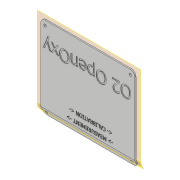
# Autodesk Inventor part: 03_Lid
Saved by Autodesk Inventor 2019.4 (Build 234330000, 330)
## iProperties
Created: 2021-06-05
Part Number: 03_Lid
Material: Generic
Document SubType Name: Modeling
Designer: diederichbenedict
Density: 1 g/cm^3
Appearance: Default
Author: diederichbenedict
Autodesk Inventor part; units mm, degrees
ref_plane "YZ Plane" through (0, 0, 0) normal (1, 0, 0) x (0, 1, 0)
ref_plane "XZ Plane" through (0, 0, 0) normal (0, 1, 0) x (-1, 0, 0)
ref_plane "XY Plane" through (0, 0, 0) normal (0, 0, 1) x (1, 0, 0)
ref_plane "Work Plane1" through (0, 0, 0) normal (0, 0, 1) x (1, 0, 0)
sketch "Sketch1" plane through (0, 0, 0) normal (0, 0, 1) x (1, 0, 0)
  ellipse E0 centre (-7.5, -84.2405) end of major axis (-7.5, -80.461) minor radius 1.5 projected
  ellipse E1 centre (-100.5, -84.2405) end of major axis (-100.5, -80.461) minor radius 1.5 projected
  ellipse E2 centre (-103, -7.7709) end of major axis (-103, -9.3506) minor radius 1.45 projected
  line L0 (-3, -61.2439) -> (-3, -12.7635) projected
  line L1 (-3, -61.2439) -> (-18, -61.2439) projected
  line L2 (-18, -90.5398) -> (-18, -61.2439) projected
  line L3 (0, -90.5398) -> (-18, -90.5398) projected
  line L4 (0, -7.7709) -> (0, -90.5398) projected
  ellipse E3 centre (-5, -7.7709) end of major axis (-5, -13.2183) minor radius 5 (0, -7.7709) -> (-5, -2.3235) ccw projected
  line L5 (-103, -2.3235) -> (-5, -2.3235) projected
  ellipse E4 centre (-103, -7.7709) end of major axis (-103, -13.2183) minor radius 5 (-103, -2.3235) -> (-108, -7.7709) ccw projected
  line L6 (-108, -90.5398) -> (-108, -7.7709) projected
  line L7 (-95, -90.5398) -> (-108, -90.5398) projected
  line L8 (-95, -61.2439) -> (-95, -90.5398) projected
  line L9 (-105, -61.2439) -> (-95, -61.2439) projected
  line L10 (-105, -12.7635) -> (-105, -61.2439) projected
  ellipse E5 centre (-103, -7.7709) end of major axis (-103, -13.2183) minor radius 5 (-105, -12.7635) -> (-98.4174, -5.5919) ccw projected
  line L11 (-9.5826, -5.5919) -> (-98.4174, -5.5919) projected
  ellipse E6 centre (-5, -7.7709) end of major axis (-5, -13.2183) minor radius 5 (-9.5826, -5.5919) -> (-3, -12.7635) ccw projected
  ellipse E7 centre (-5, -7.7709) end of major axis (-5, -9.3506) minor radius 1.45 projected
  line L12 (-18, -90.5398) -> (-95, -90.5398)
  point P0 (0, 0)
  constraints: 2 end point, 1 horizontal, 8 other
extrude "Extrusion1" add sketch "Sketch1" along normal blind 1.5 contours E0 | E1 | L1 L2 L12 L8 L9 L10 E5 L11 E6 L0 | L0 E6 L11 E5 L10 L9 L8 L7 L6 E4 L5 E3 L4 L3 L2 L1
ref_plane "Work Plane2" through (-54, -57.5226, 14.2761) normal (0, -0.3968725, 0.9178738) x (1, 0, 0)
sketch "Sketch2" plane through (-54, -57.5226, 14.2761) normal (0, -0.3968725, 0.9178738) x (1, 0, 0)
  circle A0 centre (49, -40) radius 1.45 projected
  circle A1 centre (-49, -40) radius 1.45 projected
  line L0 (-41, -35.9714) -> (-54, -35.9714) projected
  line L1 (-54, -40) -> (-54, -35.9714) projected
  arc A2 (-54, -40) -> (-49, -45) centre (-49, -40) ccw projected
  line L2 (49, -45) -> (-49, -45) projected
  arc A3 (49, -45) -> (54, -40) centre (49, -40) ccw projected
  line L3 (54, -35.9714) -> (54, -40) projected
  line L4 (54, -35.9714) -> (36, -35.9714) projected
  line L5 (36, -42) -> (36, -35.9714) projected
  line L6 (-41, -42) -> (36, -42) projected
  line L7 (-41, -35.9714) -> (-41, -42) projected
  line L8 (36, -35.9714) -> (-41, -35.9714)
  line L9 (-54, -35.9714) -> (54, -35.9714) projected
  line L10 (-54, 40) -> (-54, -35.9714) projected
  line L11 (54, -35.3761) -> (54, 40.5953) projected
  line L12 (-54, -35.9714) -> (54, -35.9714)
  line L13 (54, -35.9714) -> (54, -35.3761)
  line L14 (54, -35.3761) -> (-54, -35.3761)
  line L15 (-54, -35.3761) -> (-54, -35.9714)
  point P0 (54, 47.1327)
  constraints: 10 end point, 2 parallel, 1 collinear, 1 horizontal, 1 perpendicular
extrude "Extrusion2" add sketch "Sketch2" along normal up to surface (1.3768 mm away)
sketch "Sketch3" plane through (0, 0, 1.5) normal (0, 0, 1) x (1, 0, 0)
  ellipse E0 centre (-5, -7.7709) end of major axis (-5, -6.1911) minor radius 1.45 projected
  ellipse E1 centre (-103, -7.7709) end of major axis (-103, -6.1911) minor radius 1.45 projected
  line L0 (-108, -90.5398) -> (0, -90.5398) projected
  line L1 (0, -90.5398) -> (0, -7.7709) projected
  ellipse E2 centre (-5, -7.7709) end of major axis (-5, -13.2183) minor radius 5 (0, -7.7709) -> (-5, -2.3235) ccw projected
  line L2 (-5, -2.3235) -> (-103, -2.3235) projected
  ellipse E3 centre (-103, -7.7709) end of major axis (-103, -13.2183) minor radius 5 (-103, -2.3235) -> (-108, -7.7709) ccw projected
  line L3 (-108, -7.7709) -> (-108, -90.5398) projected
  line L4 (-3.7962, -33.7156) -> (-220.4518, -33.7156) construction
  line L5 (-220.4518, -33.7156) -> (-220.4518, 2.716) construction
  line L6 (-220.4518, 2.716) -> (-3.7962, 2.716) construction
  line L7 (-3.7962, 2.716) -> (-3.7962, -33.7156) construction
  line L8 (-24.8389, -87.8495) -> (-82.3672, -87.8495) construction
  line L9 (-82.3672, -87.8495) -> (-82.3672, -82.6215) construction
  line L10 (-82.3672, -82.6215) -> (-24.8389, -82.6215) construction
  line L11 (-24.8389, -82.6215) -> (-24.8389, -87.8495) construction
  line L12 (-25.7292, -78.9471) -> (-83.2575, -78.9471) construction
  line L13 (-83.2575, -78.9471) -> (-83.2575, -73.7191) construction
  line L14 (-83.2575, -73.7191) -> (-25.7292, -73.7191) construction
  line L15 (-25.7292, -73.7191) -> (-25.7292, -78.9471) construction
  spline S0 degree 2 poles (-14.4129, -31.9391) (-15.1575, -31.0668) (-15.9873, -28.5137) (-15.9873, -26.8754) knots 0 0 0 1 2 2 2
  spline S1 degree 2 poles (-15.9873, -26.8754) (-15.9873, -25.2798) (-15.1788, -22.6947) (-14.4129, -21.8224) knots 0 0 0 1 2 2 2
  spline S2 degree 2 poles (-14.4129, -21.8224) (-13.6044, -20.9076) (-11.4662, -20.0353) (-10.179, -20.0353) knots 0 0 0 1 2 2 2
  spline S3 degree 2 poles (-10.179, -20.0353) (-8.8492, -20.0353) (-6.7217, -20.9395) (-5.9451, -21.8224) knots 0 0 0 1 2 2 2
  spline S4 degree 2 poles (-5.9451, -21.8224) (-5.1898, -22.6947) (-4.3813, -25.2585) (-4.3813, -26.8754) knots 0 0 0 1 2 2 2
  spline S5 degree 2 poles (-4.3813, -26.8754) (-4.3813, -28.5243) (-5.2004, -31.0349) (-5.9557, -31.9391) knots 0 0 0 1 2 2 2
  spline S6 degree 2 poles (-5.9557, -31.9391) (-6.7217, -32.8114) (-8.8599, -33.7156) (-10.179, -33.7156) knots 0 0 0 1 2 2 2
  spline S7 degree 2 poles (-10.179, -33.7156) (-11.5194, -33.7156) (-13.6682, -32.7795) (-14.4129, -31.9391) knots 0 0 0 1 2 2 2
  spline S8 degree 2 poles (-14.1682, -26.8754) (-14.1682, -28.1733) (-13.6044, -30.1838) (-13.0938, -30.8434) knots 0 0 0 1 2 2 2
  spline S9 degree 2 poles (-13.0938, -30.8434) (-12.5725, -31.5242) (-11.1045, -32.205) (-10.1896, -32.205) knots 0 0 0 1 2 2 2
  spline S10 degree 2 poles (-10.1896, -32.205) (-9.2428, -32.205) (-7.8174, -31.5455) (-7.2748, -30.8434) knots 0 0 0 1 2 2 2
  spline S11 degree 2 poles (-7.2748, -30.8434) (-6.7536, -30.1732) (-6.2004, -28.152) (-6.2004, -26.8754) knots 0 0 0 1 2 2 2
  spline S12 degree 2 poles (-6.2004, -26.8754) (-6.2004, -24.2904) (-8.3705, -21.5458) (-10.1896, -21.5458) knots 0 0 0 1 2 2 2
  spline S13 degree 2 poles (-10.1896, -21.5458) (-12.0087, -21.5458) (-14.1682, -24.2904) (-14.1682, -26.8754) knots 0 0 0 1 2 2 2
  line L16 (-25.6252, -20.3118) -> (-17.5298, -20.3118)
  line L17 (-17.5298, -20.3118) -> (-17.5298, -22.1735)
  spline S14 degree 2 poles (-17.5298, -22.1735) (-18.4021, -22.9926) (-19.9552, -24.5138) (-20.6999, -25.3329) knots 0 0 0 1 2 2 2
  spline S15 degree 2 poles (-20.6999, -25.3329) (-22.1998, -26.9818) (-23.2955, -28.9605) (-23.2955, -30.0136) knots 0 0 0 1 2 2 2
  spline S16 degree 2 poles (-23.2955, -30.0136) (-23.2955, -30.5668) (-22.9551, -31.3966) (-22.6466, -31.6625) knots 0 0 0 1 2 2 2
  spline S17 degree 2 poles (-22.6466, -31.6625) (-22.3381, -31.9285) (-21.5296, -32.1944) (-21.0403, -32.1944) knots 0 0 0 1 2 2 2
  spline S18 degree 2 poles (-21.0403, -32.1944) (-20.5722, -32.1944) (-19.6148, -31.9604) (-19.1787, -31.7795) knots 0 0 0 1 2 2 2
  spline S19 degree 2 poles (-19.1787, -31.7795) (-18.8063, -31.6306) (-18.1149, -31.2051) (-17.9021, -31.0561) knots 0 0 0 1 2 2 2
  line L18 (-17.9021, -31.0561) -> (-17.8064, -31.0561)
  line L19 (-17.8064, -31.0561) -> (-17.8064, -32.9284)
  spline S20 degree 2 poles (-17.8064, -32.9284) (-18.3489, -33.1944) (-20.2956, -33.7156) (-21.168, -33.7156) knots 0 0 0 1 2 2 2
  spline S21 degree 2 poles (-21.168, -33.7156) (-23.0083, -33.7156) (-25.0827, -31.7689) (-25.0827, -30.1094) knots 0 0 0 1 2 2 2
  spline S22 degree 2 poles (-25.0827, -30.1094) (-25.0827, -29.3328) (-24.721, -28.035) (-24.4019, -27.4818) knots 0 0 0 1 2 2 2
  spline S23 degree 2 poles (-24.4019, -27.4818) (-24.0827, -26.9074) (-23.1572, -25.7797) (-22.6466, -25.2372) knots 0 0 0 1 2 2 2
  spline S24 degree 2 poles (-22.6466, -25.2372) (-21.8169, -24.333) (-19.785, -22.3969) (-19.1787, -21.8331) knots 0 0 0 1 2 2 2
  line L20 (-19.1787, -21.8331) -> (-25.6252, -21.8331)
  line L21 (-25.6252, -21.8331) -> (-25.6252, -20.3118)
  spline S25 degree 2 poles (-42.6778, -31.9391) (-43.4225, -31.0668) (-44.2523, -28.5137) (-44.2523, -26.8754) knots 0 0 0 1 2 2 2
  spline S26 degree 2 poles (-44.2523, -26.8754) (-44.2523, -25.2798) (-43.4438, -22.6947) (-42.6778, -21.8224) knots 0 0 0 1 2 2 2
  spline S27 degree 2 poles (-42.6778, -21.8224) (-41.8694, -20.9076) (-39.7311, -20.0353) (-38.4439, -20.0353) knots 0 0 0 1 2 2 2
  spline S28 degree 2 poles (-38.4439, -20.0353) (-37.1142, -20.0353) (-34.9866, -20.9395) (-34.2101, -21.8224) knots 0 0 0 1 2 2 2
  spline S29 degree 2 poles (-34.2101, -21.8224) (-33.4548, -22.6947) (-32.6463, -25.2585) (-32.6463, -26.8754) knots 0 0 0 1 2 2 2
  spline S30 degree 2 poles (-32.6463, -26.8754) (-32.6463, -28.5243) (-33.4654, -31.0349) (-34.2207, -31.9391) knots 0 0 0 1 2 2 2
  spline S31 degree 2 poles (-34.2207, -31.9391) (-34.9866, -32.8114) (-37.1248, -33.7156) (-38.4439, -33.7156) knots 0 0 0 1 2 2 2
  spline S32 degree 2 poles (-38.4439, -33.7156) (-39.7843, -33.7156) (-41.9332, -32.7795) (-42.6778, -31.9391) knots 0 0 0 1 2 2 2
  spline S33 degree 2 poles (-42.4332, -26.8754) (-42.4332, -28.1733) (-41.8694, -30.1838) (-41.3587, -30.8434) knots 0 0 0 1 2 2 2
  spline S34 degree 2 poles (-41.3587, -30.8434) (-40.8375, -31.5242) (-39.3694, -32.205) (-38.4546, -32.205) knots 0 0 0 1 2 2 2
  spline S35 degree 2 poles (-38.4546, -32.205) (-37.5078, -32.205) (-36.0823, -31.5455) (-35.5398, -30.8434) knots 0 0 0 1 2 2 2
  spline S36 degree 2 poles (-35.5398, -30.8434) (-35.0185, -30.1732) (-34.4654, -28.152) (-34.4654, -26.8754) knots 0 0 0 1 2 2 2
  spline S37 degree 2 poles (-34.4654, -26.8754) (-34.4654, -24.2904) (-36.6355, -21.5458) (-38.4546, -21.5458) knots 0 0 0 1 2 2 2
  spline S38 degree 2 poles (-38.4546, -21.5458) (-40.2737, -21.5458) (-42.4332, -24.2904) (-42.4332, -26.8754) knots 0 0 0 1 2 2 2
  spline S39 degree 2 poles (-54.2945, -25.5032) (-54.2945, -23.0352) (-51.9435, -20.1204) (-50.1457, -20.1204) knots 0 0 0 1 2 2 2
  spline S40 degree 2 poles (-50.1457, -20.1204) (-49.4116, -20.1204) (-48.284, -20.4608) (-47.6989, -20.8118) knots 0 0 0 1 2 2 2
  line L22 (-47.6989, -20.8118) -> (-47.6989, -16.6843)
  line L23 (-47.6989, -16.6843) -> (-46.0394, -16.6843)
  line L24 (-46.0394, -16.6843) -> (-46.0394, -30.1626)
  line L25 (-46.0394, -30.1626) -> (-47.6989, -30.1626)
  line L26 (-47.6989, -30.1626) -> (-47.6989, -29.1307)
  spline S41 degree 2 poles (-47.6989, -29.1307) (-48.3159, -29.6945) (-49.8265, -30.4391) (-50.7095, -30.4391) knots 0 0 0 1 2 2 2
  spline S42 degree 2 poles (-50.7095, -30.4391) (-52.4009, -30.4391) (-54.2945, -27.7584) (-54.2945, -25.5032) knots 0 0 0 1 2 2 2
  spline S43 degree 2 poles (-52.5817, -25.3117) (-52.5817, -27.0031) (-51.5073, -28.8647) (-50.3052, -28.8647) knots 0 0 0 1 2 2 2
  spline S44 degree 2 poles (-50.3052, -28.8647) (-49.6031, -28.8647) (-48.284, -28.2371) (-47.6989, -27.7478) knots 0 0 0 1 2 2 2
  line L27 (-47.6989, -27.7478) -> (-47.6989, -22.1522)
  spline S45 degree 2 poles (-47.6989, -22.1522) (-48.3479, -21.8437) (-49.2734, -21.6097) (-49.8691, -21.6097) knots 0 0 0 1 2 2 2
  spline S46 degree 2 poles (-49.8691, -21.6097) (-51.1563, -21.6097) (-52.5817, -23.5032) (-52.5817, -25.3117) knots 0 0 0 1 2 2 2
  spline S47 degree 2 poles (-60.2942, -20.0884) (-57.9326, -20.0884) (-55.337, -22.7373) (-55.337, -25.184) knots 0 0 0 1 2 2 2
  spline S48 degree 2 poles (-55.337, -25.184) (-55.337, -27.5882) (-57.8582, -30.4391) (-59.89, -30.4391) knots 0 0 0 1 2 2 2
  spline S49 degree 2 poles (-59.89, -30.4391) (-60.8049, -30.4391) (-62.2197, -29.9073) (-62.741, -29.3434) knots 0 0 0 1 2 2 2
  spline S50 degree 2 poles (-62.741, -29.3434) (-63.2729, -28.7796) (-63.8367, -27.152) (-63.8367, -25.9712) knots 0 0 0 1 2 2 2
  line L28 (-63.8367, -25.9712) -> (-63.8367, -25.067)
  line L29 (-63.8367, -25.067) -> (-57.0178, -25.067)
  spline S51 degree 2 poles (-57.0178, -25.067) (-57.0178, -23.3543) (-58.7411, -21.5352) (-60.273, -21.5352) knots 0 0 0 1 2 2 2
  spline S52 degree 2 poles (-60.273, -21.5352) (-60.8155, -21.5352) (-61.8687, -21.7799) (-62.2942, -21.9714) knots 0 0 0 1 2 2 2
  spline S53 degree 2 poles (-62.2942, -21.9714) (-62.741, -22.1841) (-63.358, -22.5564) (-63.5601, -22.7267) knots 0 0 0 1 2 2 2
  line L30 (-63.5601, -22.7267) -> (-63.6558, -22.7267)
  line L31 (-63.6558, -22.7267) -> (-63.6558, -20.9182)
  spline S54 degree 2 poles (-63.6558, -20.9182) (-63.3686, -20.8012) (-62.4963, -20.4608) (-62.1559, -20.365) knots 0 0 0 1 2 2 2
  spline S55 degree 2 poles (-62.1559, -20.365) (-61.6772, -20.2267) (-60.89, -20.0884) (-60.2942, -20.0884) knots 0 0 0 1 2 2 2
  spline S56 degree 2 poles (-62.2197, -26.3329) (-62.1984, -27.0031) (-61.9218, -27.9818) (-61.6559, -28.3116) knots 0 0 0 1 2 2 2
  spline S57 degree 2 poles (-61.6559, -28.3116) (-61.3687, -28.6839) (-60.4645, -29.0775) (-59.7943, -29.0775) knots 0 0 0 1 2 2 2
  spline S58 degree 2 poles (-59.7943, -29.0775) (-59.1347, -29.0775) (-58.2092, -28.6839) (-57.8262, -28.3009) knots 0 0 0 1 2 2 2
  spline S59 degree 2 poles (-57.8262, -28.3009) (-57.4539, -27.9073) (-57.071, -26.9605) (-57.0178, -26.3329) knots 0 0 0 1 2 2 2
  line L32 (-57.0178, -26.3329) -> (-62.2197, -26.3329)
  line L33 (-73.2512, -20.3118) -> (-71.5917, -20.3118)
  line L34 (-71.5917, -20.3118) -> (-71.5917, -25.9287)
  spline S60 degree 2 poles (-71.5917, -25.9287) (-71.5917, -26.6095) (-71.4641, -27.7797) (-71.2726, -28.1307) knots 0 0 0 1 2 2 2
  spline S61 degree 2 poles (-71.2726, -28.1307) (-71.0705, -28.503) (-70.3471, -28.8647) (-69.7301, -28.8647) knots 0 0 0 1 2 2 2
  spline S62 degree 2 poles (-69.7301, -28.8647) (-69.1131, -28.8647) (-67.8046, -28.2052) (-67.177, -27.6733) knots 0 0 0 1 2 2 2
  line L35 (-67.177, -27.6733) -> (-67.177, -20.3118)
  line L36 (-67.177, -20.3118) -> (-65.5175, -20.3118)
  line L37 (-65.5175, -20.3118) -> (-65.5175, -30.1626)
  line L38 (-65.5175, -30.1626) -> (-67.177, -30.1626)
  line L39 (-67.177, -30.1626) -> (-67.177, -29.0669)
  spline S63 degree 2 poles (-67.177, -29.0669) (-67.9216, -29.737) (-69.3578, -30.4391) (-70.1662, -30.4391) knots 0 0 0 1 2 2 2
  spline S64 degree 2 poles (-70.1662, -30.4391) (-71.613, -30.4391) (-73.2512, -28.5243) (-73.2512, -26.7052) knots 0 0 0 1 2 2 2
  line L40 (-73.2512, -26.7052) -> (-73.2512, -20.3118)
  spline S65 degree 2 poles (-84.9955, -31.9391) (-85.7402, -31.0668) (-86.5699, -28.5137) (-86.5699, -26.8754) knots 0 0 0 1 2 2 2
  spline S66 degree 2 poles (-86.5699, -26.8754) (-86.5699, -25.2798) (-85.7614, -22.6947) (-84.9955, -21.8224) knots 0 0 0 1 2 2 2
  spline S67 degree 2 poles (-84.9955, -21.8224) (-84.187, -20.9076) (-82.0488, -20.0353) (-80.7616, -20.0353) knots 0 0 0 1 2 2 2
  spline S68 degree 2 poles (-80.7616, -20.0353) (-79.4319, -20.0353) (-77.3043, -20.9395) (-76.5277, -21.8224) knots 0 0 0 1 2 2 2
  spline S69 degree 2 poles (-76.5277, -21.8224) (-75.7724, -22.6947) (-74.9639, -25.2585) (-74.9639, -26.8754) knots 0 0 0 1 2 2 2
  spline S70 degree 2 poles (-74.9639, -26.8754) (-74.9639, -28.5243) (-75.7831, -31.0349) (-76.5384, -31.9391) knots 0 0 0 1 2 2 2
  spline S71 degree 2 poles (-76.5384, -31.9391) (-77.3043, -32.8114) (-79.4425, -33.7156) (-80.7616, -33.7156) knots 0 0 0 1 2 2 2
  spline S72 degree 2 poles (-80.7616, -33.7156) (-82.102, -33.7156) (-84.2509, -32.7795) (-84.9955, -31.9391) knots 0 0 0 1 2 2 2
  spline S73 degree 2 poles (-84.7508, -26.8754) (-84.7508, -28.1733) (-84.187, -30.1838) (-83.6764, -30.8434) knots 0 0 0 1 2 2 2
  spline S74 degree 2 poles (-83.6764, -30.8434) (-83.1551, -31.5242) (-81.6871, -32.205) (-80.7723, -32.205) knots 0 0 0 1 2 2 2
  spline S75 degree 2 poles (-80.7723, -32.205) (-79.8255, -32.205) (-78.4, -31.5455) (-77.8575, -30.8434) knots 0 0 0 1 2 2 2
  spline S76 degree 2 poles (-77.8575, -30.8434) (-77.3362, -30.1732) (-76.783, -28.152) (-76.783, -26.8754) knots 0 0 0 1 2 2 2
  spline S77 degree 2 poles (-76.783, -26.8754) (-76.783, -24.2904) (-78.9532, -21.5458) (-80.7723, -21.5458) knots 0 0 0 1 2 2 2
  spline S78 degree 2 poles (-80.7723, -21.5458) (-82.5913, -21.5458) (-84.7508, -24.2904) (-84.7508, -26.8754) knots 0 0 0 1 2 2 2
  line L41 (-96.0058, -20.3118) -> (-93.9739, -20.3118)
  line L42 (-93.9739, -20.3118) -> (-91.5804, -24.0138)
  line L43 (-91.5804, -24.0138) -> (-89.123, -20.3118)
  line L44 (-89.123, -20.3118) -> (-87.2401, -20.3118)
  line L45 (-87.2401, -20.3118) -> (-90.6549, -25.1947)
  line L46 (-90.6549, -25.1947) -> (-87.272, -30.1626)
  line L47 (-87.272, -30.1626) -> (-89.3039, -30.1626)
  line L48 (-89.3039, -30.1626) -> (-91.6868, -26.4925)
  line L49 (-91.6868, -26.4925) -> (-94.1228, -30.1626)
  line L50 (-94.1228, -30.1626) -> (-96.0058, -30.1626)
  line L51 (-96.0058, -30.1626) -> (-92.6123, -25.301)
  line L52 (-92.6123, -25.301) -> (-96.0058, -20.3118)
  line L53 (-105.0267, -30.1626) -> (-99.729, -16.6843)
  line L54 (-99.729, -16.6843) -> (-97.9525, -16.6843)
  line L55 (-97.9525, -16.6843) -> (-99.7184, -20.7906)
  line L56 (-99.7184, -20.7906) -> (-96.1441, -30.1626)
  line L57 (-96.1441, -30.1626) -> (-97.9312, -30.1626)
  line L58 (-97.9312, -30.1626) -> (-100.6226, -22.8649)
  line L59 (-100.6226, -22.8649) -> (-103.3034, -30.1626)
  line L60 (-103.3034, -30.1626) -> (-105.0267, -30.1626)
  line L61 (-29.1554, -75.0735) -> (-26.2705, -76.4512)
  line L62 (-26.2705, -76.4512) -> (-26.2705, -76.7721)
  line L63 (-26.2705, -76.7721) -> (-29.1554, -78.1497)
  line L64 (-29.1554, -78.1497) -> (-29.1554, -77.6732)
  line L65 (-29.1554, -77.6732) -> (-26.9188, -76.6132)
  line L66 (-26.9188, -76.6132) -> (-29.1554, -75.55)
  line L67 (-29.1554, -75.55) -> (-29.1554, -75.0735)
  line L68 (-31.4893, -76.3701) -> (-29.9755, -76.3701)
  line L69 (-29.9755, -76.3701) -> (-29.9755, -76.8564)
  line L70 (-29.9755, -76.8564) -> (-31.4893, -76.8564)
  line L71 (-31.4893, -76.8564) -> (-31.4893, -76.3701)
  spline S79 degree 2 poles (-35.4147, -74.7915) (-35.0257, -74.7915) (-34.3677, -75.0541) (-34.1279, -75.3167) knots 0 0 0 1 2 2 2
  spline S80 degree 2 poles (-34.1279, -75.3167) (-33.888, -75.576) (-33.6254, -76.3539) (-33.6254, -76.8596) knots 0 0 0 1 2 2 2
  spline S81 degree 2 poles (-33.6254, -76.8596) (-33.6254, -77.362) (-33.8815, -78.1076) (-34.1246, -78.3831) knots 0 0 0 1 2 2 2
  spline S82 degree 2 poles (-34.1246, -78.3831) (-34.3645, -78.6521) (-35.0193, -78.9342) (-35.4245, -78.9342) knots 0 0 0 1 2 2 2
  spline S83 degree 2 poles (-35.4245, -78.9342) (-35.6254, -78.9342) (-35.9787, -78.8758) (-36.1279, -78.8304) knots 0 0 0 1 2 2 2
  spline S84 degree 2 poles (-36.1279, -78.8304) (-36.2575, -78.7883) (-36.5266, -78.6684) (-36.6595, -78.597) knots 0 0 0 1 2 2 2
  line L72 (-36.6595, -78.597) -> (-36.6595, -77.9552)
  line L73 (-36.6595, -77.9552) -> (-36.6173, -77.9552)
  spline S85 degree 2 poles (-36.6173, -77.9552) (-36.546, -78.0201) (-36.3256, -78.2016) (-36.1668, -78.2891) knots 0 0 0 1 2 2 2
  spline S86 degree 2 poles (-36.1668, -78.2891) (-36.0144, -78.3734) (-35.6546, -78.4803) (-35.4212, -78.4803) knots 0 0 0 1 2 2 2
  spline S87 degree 2 poles (-35.4212, -78.4803) (-35.1651, -78.4803) (-34.7081, -78.2697) (-34.5363, -78.0687) knots 0 0 0 1 2 2 2
  spline S88 degree 2 poles (-34.5363, -78.0687) (-34.3677, -77.8645) (-34.1797, -77.2453) (-34.1797, -76.8596) knots 0 0 0 1 2 2 2
  spline S89 degree 2 poles (-34.1797, -76.8596) (-34.1797, -76.4479) (-34.3774, -75.8547) (-34.5492, -75.6505) knots 0 0 0 1 2 2 2
  spline S90 degree 2 poles (-34.5492, -75.6505) (-34.7178, -75.4528) (-35.1684, -75.2518) (-35.4212, -75.2518) knots 0 0 0 1 2 2 2
  spline S91 degree 2 poles (-35.4212, -75.2518) (-35.6514, -75.2518) (-36.0436, -75.3653) (-36.1959, -75.4496) knots 0 0 0 1 2 2 2
  spline S92 degree 2 poles (-36.1959, -75.4496) (-36.3418, -75.5338) (-36.559, -75.7089) (-36.6206, -75.7705) knots 0 0 0 1 2 2 2
  line L74 (-36.6206, -75.7705) -> (-36.6595, -75.7705)
  line L75 (-36.6595, -75.7705) -> (-36.6595, -75.1351)
  spline S93 degree 2 poles (-36.6595, -75.1351) (-36.5266, -75.0735) (-36.2932, -74.9601) (-36.1279, -74.9082) knots 0 0 0 1 2 2 2
  spline S94 degree 2 poles (-36.1279, -74.9082) (-35.9528, -74.8499) (-35.6546, -74.7915) (-35.4147, -74.7915) knots 0 0 0 1 2 2 2
  line L76 (-36.7243, -74.8628) -> (-38.0727, -78.8628)
  line L77 (-38.0727, -78.8628) -> (-38.7275, -78.8628)
  line L78 (-38.7275, -78.8628) -> (-40.076, -74.8628)
  line L79 (-40.076, -74.8628) -> (-39.5152, -74.8628)
  line L80 (-39.5152, -74.8628) -> (-39.1522, -75.9812)
  line L81 (-39.1522, -75.9812) -> (-37.6254, -75.9812)
  line L82 (-37.6254, -75.9812) -> (-37.2624, -74.8628)
  line L83 (-37.2624, -74.8628) -> (-36.7243, -74.8628)
  line L84 (-39.0063, -76.435) -> (-38.3872, -78.3183)
  line L85 (-38.3872, -78.3183) -> (-37.7713, -76.435)
  line L86 (-37.7713, -76.435) -> (-39.0063, -76.435)
  line L87 (-42.7729, -74.8628) -> (-40.4552, -74.8628)
  line L88 (-40.4552, -74.8628) -> (-40.4552, -78.8628)
  line L89 (-40.4552, -78.8628) -> (-40.9869, -78.8628)
  line L90 (-40.9869, -78.8628) -> (-40.9869, -75.3361)
  line L91 (-40.9869, -75.3361) -> (-42.7729, -75.3361)
  line L92 (-42.7729, -75.3361) -> (-42.7729, -74.8628)
  line L93 (-44.5849, -74.8628) -> (-43.0355, -74.8628)
  line L94 (-43.0355, -74.8628) -> (-43.0355, -75.2713)
  line L95 (-43.0355, -75.2713) -> (-43.5444, -75.2713)
  line L96 (-43.5444, -75.2713) -> (-43.5444, -78.4544)
  line L97 (-43.5444, -78.4544) -> (-43.0355, -78.4544)
  line L98 (-43.0355, -78.4544) -> (-43.0355, -78.8628)
  line L99 (-43.0355, -78.8628) -> (-44.5849, -78.8628)
  line L100 (-44.5849, -78.8628) -> (-44.5849, -78.4544)
  line L101 (-44.5849, -78.4544) -> (-44.076, -78.4544)
  line L102 (-44.076, -78.4544) -> (-44.076, -75.2713)
  line L103 (-44.076, -75.2713) -> (-44.5849, -75.2713)
  line L104 (-44.5849, -75.2713) -> (-44.5849, -74.8628)
  spline S95 degree 2 poles (-47.9561, -76.0914) (-47.9561, -75.7932) (-47.7292, -75.3361) (-47.5411, -75.187) knots 0 0 0 1 2 2 2
  spline S96 degree 2 poles (-47.5411, -75.187) (-47.3142, -75.012) (-46.7988, -74.8628) (-46.3904, -74.8628) knots 0 0 0 1 2 2 2
  line L105 (-46.3904, -74.8628) -> (-45.2429, -74.8628)
  line L106 (-45.2429, -74.8628) -> (-45.2429, -78.8628)
  line L107 (-45.2429, -78.8628) -> (-46.3029, -78.8628)
  spline S97 degree 2 poles (-46.3029, -78.8628) (-46.7308, -78.8628) (-47.1586, -78.8077) (-47.3531, -78.7008) knots 0 0 0 1 2 2 2
  spline S98 degree 2 poles (-47.3531, -78.7008) (-47.5703, -78.5873) (-47.768, -78.2145) (-47.768, -77.9617) knots 0 0 0 1 2 2 2
  spline S99 degree 2 poles (-47.768, -77.9617) (-47.768, -77.6797) (-47.4698, -77.2324) (-47.2073, -77.106) knots 0 0 0 1 2 2 2
  line L108 (-47.2073, -77.106) -> (-47.2073, -77.0865)
  spline S100 degree 2 poles (-47.2073, -77.0865) (-47.5638, -76.9893) (-47.9561, -76.4739) (-47.9561, -76.0914) knots 0 0 0 1 2 2 2
  spline S101 degree 2 poles (-47.4018, -76.0687) (-47.4018, -76.2956) (-47.2721, -76.5873) (-47.0776, -76.691) knots 0 0 0 1 2 2 2
  spline S102 degree 2 poles (-47.0776, -76.691) (-46.9512, -76.7559) (-46.653, -76.7948) (-46.3774, -76.7948) knots 0 0 0 1 2 2 2
  line L109 (-46.3774, -76.7948) -> (-45.7745, -76.7948)
  line L110 (-45.7745, -76.7948) -> (-45.7745, -75.3167)
  line L111 (-45.7745, -75.3167) -> (-46.2057, -75.3167)
  spline S103 degree 2 poles (-46.2057, -75.3167) (-46.5557, -75.3167) (-46.9577, -75.3815) (-47.1133, -75.4852) knots 0 0 0 1 2 2 2
  spline S104 degree 2 poles (-47.1133, -75.4852) (-47.2624, -75.5922) (-47.4018, -75.858) (-47.4018, -76.0687) knots 0 0 0 1 2 2 2
  spline S105 degree 2 poles (-47.2138, -77.8872) (-47.2138, -78.0298) (-47.1165, -78.2437) (-47.0095, -78.3053) knots 0 0 0 1 2 2 2
  spline S106 degree 2 poles (-47.0095, -78.3053) (-46.8799, -78.3766) (-46.5655, -78.409) (-46.2834, -78.409) knots 0 0 0 1 2 2 2
  line L112 (-46.2834, -78.409) -> (-45.7745, -78.409)
  line L113 (-45.7745, -78.409) -> (-45.7745, -77.2389)
  line L114 (-45.7745, -77.2389) -> (-46.3774, -77.2389)
  spline S107 degree 2 poles (-46.3774, -77.2389) (-46.627, -77.2389) (-46.8637, -77.2907) (-46.9901, -77.3718) knots 0 0 0 1 2 2 2
  spline S108 degree 2 poles (-46.9901, -77.3718) (-47.1133, -77.4496) (-47.2138, -77.6991) (-47.2138, -77.8872) knots 0 0 0 1 2 2 2
  line L115 (-51.58, -74.8628) -> (-50.8896, -74.8628)
  line L116 (-50.8896, -74.8628) -> (-49.6254, -76.4544)
  line L117 (-49.6254, -76.4544) -> (-49.016, -76.4544)
  line L118 (-49.016, -76.4544) -> (-49.016, -74.8628)
  line L119 (-49.016, -74.8628) -> (-48.4844, -74.8628)
  line L120 (-48.4844, -74.8628) -> (-48.4844, -78.8628)
  line L121 (-48.4844, -78.8628) -> (-49.5152, -78.8628)
  spline S109 degree 2 poles (-49.5152, -78.8628) (-49.8588, -78.8628) (-50.3223, -78.7883) (-50.533, -78.6521) knots 0 0 0 1 2 2 2
  spline S110 degree 2 poles (-50.533, -78.6521) (-50.7437, -78.516) (-50.9869, -78.0914) (-50.9869, -77.7769) knots 0 0 0 1 2 2 2
  spline S111 degree 2 poles (-50.9869, -77.7769) (-50.9869, -77.3393) (-50.5395, -76.7461) (-50.157, -76.6035) knots 0 0 0 1 2 2 2
  line L122 (-50.157, -76.6035) -> (-51.58, -74.8628)
  spline S112 degree 2 poles (-50.4326, -77.7348) (-50.4326, -77.9098) (-50.3094, -78.1789) (-50.1797, -78.2664) knots 0 0 0 1 2 2 2
  spline S113 degree 2 poles (-50.1797, -78.2664) (-50.0663, -78.341) (-49.7648, -78.4026) (-49.5444, -78.4026) knots 0 0 0 1 2 2 2
  line L123 (-49.5444, -78.4026) -> (-49.016, -78.4026)
  line L124 (-49.016, -78.4026) -> (-49.016, -76.8985)
  line L125 (-49.016, -76.8985) -> (-49.4828, -76.8985)
  spline S114 degree 2 poles (-49.4828, -76.8985) (-49.7129, -76.8985) (-50.0792, -76.9795) (-50.2057, -77.106) knots 0 0 0 1 2 2 2
  spline S115 degree 2 poles (-50.2057, -77.106) (-50.3223, -77.2162) (-50.4326, -77.5273) (-50.4326, -77.7348) knots 0 0 0 1 2 2 2
  line L126 (-51.4666, -74.8628) -> (-52.8151, -78.8628)
  line L127 (-52.8151, -78.8628) -> (-53.4698, -78.8628)
  line L128 (-53.4698, -78.8628) -> (-54.8183, -74.8628)
  line L129 (-54.8183, -74.8628) -> (-54.2575, -74.8628)
  line L130 (-54.2575, -74.8628) -> (-53.8945, -75.9812)
  line L131 (-53.8945, -75.9812) -> (-52.3677, -75.9812)
  line L132 (-52.3677, -75.9812) -> (-52.0047, -74.8628)
  line L133 (-52.0047, -74.8628) -> (-51.4666, -74.8628)
  line L134 (-53.7486, -76.435) -> (-53.1295, -78.3183)
  line L135 (-53.1295, -78.3183) -> (-52.5136, -76.435)
  line L136 (-52.5136, -76.435) -> (-53.7486, -76.435)
  line L137 (-56.1311, -74.8628) -> (-56.1311, -78.3896)
  line L138 (-56.1311, -78.3896) -> (-54.7891, -78.3896)
  line L139 (-54.7891, -78.3896) -> (-54.7891, -78.8628)
  line L140 (-54.7891, -78.8628) -> (-58.0047, -78.8628)
  line L141 (-58.0047, -78.8628) -> (-58.0047, -78.3896)
  line L142 (-58.0047, -78.3896) -> (-56.6627, -78.3896)
  line L143 (-56.6627, -78.3896) -> (-56.6627, -74.8628)
  line L144 (-56.6627, -74.8628) -> (-56.1311, -74.8628)
  line L145 (-59.8037, -74.8628) -> (-58.2543, -74.8628)
  line L146 (-58.2543, -74.8628) -> (-58.2543, -75.2713)
  line L147 (-58.2543, -75.2713) -> (-58.7632, -75.2713)
  line L148 (-58.7632, -75.2713) -> (-58.7632, -78.4544)
  line L149 (-58.7632, -78.4544) -> (-58.2543, -78.4544)
  line L150 (-58.2543, -78.4544) -> (-58.2543, -78.8628)
  line L151 (-58.2543, -78.8628) -> (-59.8037, -78.8628)
  line L152 (-59.8037, -78.8628) -> (-59.8037, -78.4544)
  line L153 (-59.8037, -78.4544) -> (-59.2948, -78.4544)
  line L154 (-59.2948, -78.4544) -> (-59.2948, -75.2713)
  line L155 (-59.2948, -75.2713) -> (-59.8037, -75.2713)
  line L156 (-59.8037, -75.2713) -> (-59.8037, -74.8628)
  spline S116 degree 2 poles (-63.2916, -78.4058) (-63.5185, -78.14) (-63.7713, -77.362) (-63.7713, -76.8628) knots 0 0 0 1 2 2 2
  spline S117 degree 2 poles (-63.7713, -76.8628) (-63.7713, -76.3766) (-63.5249, -75.5889) (-63.2916, -75.3231) knots 0 0 0 1 2 2 2
  spline S118 degree 2 poles (-63.2916, -75.3231) (-63.0452, -75.0444) (-62.3937, -74.7786) (-62.0014, -74.7786) knots 0 0 0 1 2 2 2
  spline S119 degree 2 poles (-62.0014, -74.7786) (-61.5963, -74.7786) (-60.948, -75.0541) (-60.7113, -75.3231) knots 0 0 0 1 2 2 2
  spline S120 degree 2 poles (-60.7113, -75.3231) (-60.4812, -75.5889) (-60.2348, -76.3701) (-60.2348, -76.8628) knots 0 0 0 1 2 2 2
  spline S121 degree 2 poles (-60.2348, -76.8628) (-60.2348, -77.3653) (-60.4844, -78.1303) (-60.7146, -78.4058) knots 0 0 0 1 2 2 2
  spline S122 degree 2 poles (-60.7146, -78.4058) (-60.948, -78.6716) (-61.5995, -78.9471) (-62.0014, -78.9471) knots 0 0 0 1 2 2 2
  spline S123 degree 2 poles (-62.0014, -78.9471) (-62.4099, -78.9471) (-63.0646, -78.6619) (-63.2916, -78.4058) knots 0 0 0 1 2 2 2
  spline S124 degree 2 poles (-63.217, -76.8628) (-63.217, -77.2583) (-63.0452, -77.8709) (-62.8896, -78.0719) knots 0 0 0 1 2 2 2
  spline S125 degree 2 poles (-62.8896, -78.0719) (-62.7308, -78.2794) (-62.2834, -78.4868) (-62.0047, -78.4868) knots 0 0 0 1 2 2 2
  spline S126 degree 2 poles (-62.0047, -78.4868) (-61.7162, -78.4868) (-61.2818, -78.2859) (-61.1165, -78.0719) knots 0 0 0 1 2 2 2
  spline S127 degree 2 poles (-61.1165, -78.0719) (-60.9577, -77.8677) (-60.7891, -77.2518) (-60.7891, -76.8628) knots 0 0 0 1 2 2 2
  spline S128 degree 2 poles (-60.7891, -76.8628) (-60.7891, -76.0752) (-61.4504, -75.2389) (-62.0047, -75.2389) knots 0 0 0 1 2 2 2
  spline S129 degree 2 poles (-62.0047, -75.2389) (-62.559, -75.2389) (-63.217, -76.0752) (-63.217, -76.8628) knots 0 0 0 1 2 2 2
  line L157 (-67.217, -74.8628) -> (-66.6206, -74.8628)
  line L158 (-66.6206, -74.8628) -> (-64.8507, -78.3118)
  line L159 (-64.8507, -78.3118) -> (-64.8507, -74.8628)
  line L160 (-64.8507, -74.8628) -> (-64.3548, -74.8628)
  line L161 (-64.3548, -74.8628) -> (-64.3548, -78.8628)
  line L162 (-64.3548, -78.8628) -> (-65.11, -78.8628)
  line L163 (-65.11, -78.8628) -> (-66.721, -75.6959)
  line L164 (-66.721, -75.6959) -> (-66.721, -78.8628)
  line L165 (-66.721, -78.8628) -> (-67.217, -78.8628)
  line L166 (-67.217, -78.8628) -> (-67.217, -74.8628)
  line L167 (-72.7664, -75.0735) -> (-69.8815, -76.4512)
  line L168 (-69.8815, -76.4512) -> (-69.8815, -76.7721)
  line L169 (-69.8815, -76.7721) -> (-72.7664, -78.1497)
  line L170 (-72.7664, -78.1497) -> (-72.7664, -77.6732)
  line L171 (-72.7664, -77.6732) -> (-70.5298, -76.6132)
  line L172 (-70.5298, -76.6132) -> (-72.7664, -75.55)
  line L173 (-72.7664, -75.55) -> (-72.7664, -75.0735)
  line L174 (-75.1003, -76.3701) -> (-73.5865, -76.3701)
  line L175 (-73.5865, -76.3701) -> (-73.5865, -76.8564)
  line L176 (-73.5865, -76.8564) -> (-75.1003, -76.8564)
  line L177 (-75.1003, -76.8564) -> (-75.1003, -76.3701)
  line L178 (-26.5958, -85.2855) -> (-25.082, -85.2855)
  line L179 (-25.082, -85.2855) -> (-25.082, -85.7717)
  line L180 (-25.082, -85.7717) -> (-26.5958, -85.7717)
  line L181 (-26.5958, -85.7717) -> (-26.5958, -85.2855)
  line L182 (-30.2976, -85.3665) -> (-27.4127, -83.9889)
  line L183 (-27.4127, -83.9889) -> (-27.4127, -84.4654)
  line L184 (-27.4127, -84.4654) -> (-29.6493, -85.5286)
  line L185 (-29.6493, -85.5286) -> (-27.4127, -86.5886)
  line L186 (-27.4127, -86.5886) -> (-27.4127, -87.0651)
  line L187 (-27.4127, -87.0651) -> (-30.2976, -85.6874)
  line L188 (-30.2976, -85.6874) -> (-30.2976, -85.3665)
  line L189 (-36.3916, -83.7782) -> (-35.86, -83.7782)
  line L190 (-35.86, -83.7782) -> (-35.86, -87.2239)
  line L191 (-35.86, -87.2239) -> (-34.8162, -84.8803)
  line L192 (-34.8162, -84.8803) -> (-34.4921, -84.8803)
  line L193 (-34.4921, -84.8803) -> (-33.458, -87.2239)
  line L194 (-33.458, -87.2239) -> (-33.458, -83.7782)
  line L195 (-33.458, -83.7782) -> (-32.9621, -83.7782)
  line L196 (-32.9621, -83.7782) -> (-32.9621, -87.7782)
  line L197 (-32.9621, -87.7782) -> (-33.6882, -87.7782)
  line L198 (-33.6882, -87.7782) -> (-34.6866, -85.5513)
  line L199 (-34.6866, -85.5513) -> (-35.6525, -87.7782)
  line L200 (-35.6525, -87.7782) -> (-36.3916, -87.7782)
  line L201 (-36.3916, -87.7782) -> (-36.3916, -83.7782)
  line L202 (-37.202, -83.7782) -> (-37.202, -87.7782)
  line L203 (-37.202, -87.7782) -> (-39.7044, -87.7782)
  line L204 (-39.7044, -87.7782) -> (-39.7044, -87.305)
  line L205 (-39.7044, -87.305) -> (-37.7336, -87.305)
  line L206 (-37.7336, -87.305) -> (-37.7336, -86.2093)
  line L207 (-37.7336, -86.2093) -> (-39.5715, -86.2093)
  line L208 (-39.5715, -86.2093) -> (-39.5715, -85.7361)
  line L209 (-39.5715, -85.7361) -> (-37.7336, -85.7361)
  line L210 (-37.7336, -85.7361) -> (-37.7336, -84.2515)
  line L211 (-37.7336, -84.2515) -> (-39.7044, -84.2515)
  line L212 (-39.7044, -84.2515) -> (-39.7044, -83.7782)
  line L213 (-39.7044, -83.7782) -> (-37.202, -83.7782)
  line L214 (-39.8567, -83.7782) -> (-41.2052, -87.7782)
  line L215 (-41.2052, -87.7782) -> (-41.86, -87.7782)
  line L216 (-41.86, -87.7782) -> (-43.2084, -83.7782)
  line L217 (-43.2084, -83.7782) -> (-42.6477, -83.7782)
  line L218 (-42.6477, -83.7782) -> (-42.2846, -84.8965)
  line L219 (-42.2846, -84.8965) -> (-40.7579, -84.8965)
  line L220 (-40.7579, -84.8965) -> (-40.3948, -83.7782)
  line L221 (-40.3948, -83.7782) -> (-39.8567, -83.7782)
  line L222 (-42.1387, -85.3503) -> (-41.5196, -87.2336)
  line L223 (-41.5196, -87.2336) -> (-40.9037, -85.3503)
  line L224 (-40.9037, -85.3503) -> (-42.1387, -85.3503)
  spline S130 degree 2 poles (-44.7028, -83.7069) (-44.2684, -83.7069) (-43.659, -83.8884) (-43.39, -84.0181) knots 0 0 0 1 2 2 2
  line L225 (-43.39, -84.0181) -> (-43.39, -84.6858)
  line L226 (-43.39, -84.6858) -> (-43.4289, -84.6858)
  spline S131 degree 2 poles (-43.4289, -84.6858) (-43.6914, -84.4395) (-44.3559, -84.1672) (-44.6639, -84.1672) knots 0 0 0 1 2 2 2
  spline S132 degree 2 poles (-44.6639, -84.1672) (-45.1047, -84.1672) (-45.5553, -84.5335) (-45.5553, -84.8349) knots 0 0 0 1 2 2 2
  spline S133 degree 2 poles (-45.5553, -84.8349) (-45.5553, -85.0748) (-45.3187, -85.373) (-45.0626, -85.4476) knots 0 0 0 1 2 2 2
  spline S134 degree 2 poles (-45.0626, -85.4476) (-44.8778, -85.4994) (-44.5699, -85.5708) (-44.3397, -85.6291) knots 0 0 0 1 2 2 2
  spline S135 degree 2 poles (-44.3397, -85.6291) (-44.1323, -85.6842) (-43.8049, -85.8495) (-43.6785, -85.9824) knots 0 0 0 1 2 2 2
  spline S136 degree 2 poles (-43.6785, -85.9824) (-43.5553, -86.1153) (-43.4191, -86.4719) (-43.4191, -86.7053) knots 0 0 0 1 2 2 2
  spline S137 degree 2 poles (-43.4191, -86.7053) (-43.4191, -87.1915) (-44.1776, -87.8495) (-44.7644, -87.8495) knots 0 0 0 1 2 2 2
  spline S138 degree 2 poles (-44.7644, -87.8495) (-45.1015, -87.8495) (-45.6979, -87.7166) (-45.954, -87.5902) knots 0 0 0 1 2 2 2
  line L227 (-45.954, -87.5902) -> (-45.954, -86.9549)
  line L228 (-45.954, -86.9549) -> (-45.9151, -86.9549)
  spline S139 degree 2 poles (-45.9151, -86.9549) (-45.7238, -87.1299) (-45.1274, -87.3892) (-44.8, -87.3892) knots 0 0 0 1 2 2 2
  spline S140 degree 2 poles (-44.8, -87.3892) (-44.4305, -87.3892) (-43.9734, -87.0424) (-43.9734, -86.7604) knots 0 0 0 1 2 2 2
  spline S141 degree 2 poles (-43.9734, -86.7604) (-43.9734, -86.5075) (-44.2425, -86.2061) (-44.4953, -86.138) knots 0 0 0 1 2 2 2
  spline S142 degree 2 poles (-44.4953, -86.138) (-44.6639, -86.0926) (-45.1533, -85.9759) (-45.3154, -85.9273) knots 0 0 0 1 2 2 2
  spline S143 degree 2 poles (-45.3154, -85.9273) (-45.7271, -85.8009) (-46.1096, -85.292) (-46.1096, -84.9192) knots 0 0 0 1 2 2 2
  spline S144 degree 2 poles (-46.1096, -84.9192) (-46.1096, -84.6826) (-45.9183, -84.2288) (-45.7465, -84.0699) knots 0 0 0 1 2 2 2
  spline S145 degree 2 poles (-45.7465, -84.0699) (-45.5553, -83.8949) (-45.0691, -83.7069) (-44.7028, -83.7069) knots 0 0 0 1 2 2 2
  spline S146 degree 2 poles (-48.048, -83.6939) (-47.6947, -83.6939) (-47.1695, -83.8787) (-46.9848, -84.0635) knots 0 0 0 1 2 2 2
  spline S147 degree 2 poles (-46.9848, -84.0635) (-46.7741, -84.2709) (-46.6023, -84.8544) (-46.6023, -85.2823) knots 0 0 0 1 2 2 2
  line L229 (-46.6023, -85.2823) -> (-46.6023, -87.7782)
  line L230 (-46.6023, -87.7782) -> (-47.1339, -87.7782)
  line L231 (-47.1339, -87.7782) -> (-47.1339, -85.2823)
  spline S148 degree 2 poles (-47.1339, -85.2823) (-47.1339, -85.0035) (-47.2052, -84.6275) (-47.3057, -84.4751) knots 0 0 0 1 2 2 2
  spline S149 degree 2 poles (-47.3057, -84.4751) (-47.4127, -84.3131) (-47.7822, -84.1477) (-48.048, -84.1477) knots 0 0 0 1 2 2 2
  spline S150 degree 2 poles (-48.048, -84.1477) (-48.2976, -84.1477) (-48.6866, -84.3131) (-48.7935, -84.4751) knots 0 0 0 1 2 2 2
  spline S151 degree 2 poles (-48.7935, -84.4751) (-48.894, -84.6275) (-48.9653, -85.0003) (-48.9653, -85.2693) knots 0 0 0 1 2 2 2
  line L232 (-48.9653, -85.2693) -> (-48.9653, -87.7782)
  line L233 (-48.9653, -87.7782) -> (-49.4969, -87.7782)
  line L234 (-49.4969, -87.7782) -> (-49.4969, -85.2823)
  spline S152 degree 2 poles (-49.4969, -85.2823) (-49.4969, -84.8641) (-49.3284, -84.2677) (-49.1144, -84.0635) knots 0 0 0 1 2 2 2
  spline S153 degree 2 poles (-49.1144, -84.0635) (-48.9232, -83.8755) (-48.4175, -83.6939) (-48.048, -83.6939) knots 0 0 0 1 2 2 2
  line L235 (-53.3543, -83.7782) -> (-52.6639, -83.7782)
  line L236 (-52.6639, -83.7782) -> (-51.3997, -85.3698)
  line L237 (-51.3997, -85.3698) -> (-50.7903, -85.3698)
  line L238 (-50.7903, -85.3698) -> (-50.7903, -83.7782)
  line L239 (-50.7903, -83.7782) -> (-50.2587, -83.7782)
  line L240 (-50.2587, -83.7782) -> (-50.2587, -87.7782)
  line L241 (-50.2587, -87.7782) -> (-51.2895, -87.7782)
  spline S154 degree 2 poles (-51.2895, -87.7782) (-51.6331, -87.7782) (-52.0966, -87.7037) (-52.3073, -87.5675) knots 0 0 0 1 2 2 2
  spline S155 degree 2 poles (-52.3073, -87.5675) (-52.518, -87.4314) (-52.7611, -87.0067) (-52.7611, -86.6923) knots 0 0 0 1 2 2 2
  spline S156 degree 2 poles (-52.7611, -86.6923) (-52.7611, -86.2547) (-52.3138, -85.6615) (-51.9313, -85.5189) knots 0 0 0 1 2 2 2
  line L242 (-51.9313, -85.5189) -> (-53.3543, -83.7782)
  spline S157 degree 2 poles (-52.2068, -86.6502) (-52.2068, -86.8252) (-52.0836, -87.0943) (-51.954, -87.1818) knots 0 0 0 1 2 2 2
  spline S158 degree 2 poles (-51.954, -87.1818) (-51.8405, -87.2563) (-51.5391, -87.3179) (-51.3187, -87.3179) knots 0 0 0 1 2 2 2
  line L243 (-51.3187, -87.3179) -> (-50.7903, -87.3179)
  line L244 (-50.7903, -87.3179) -> (-50.7903, -85.8139)
  line L245 (-50.7903, -85.8139) -> (-51.2571, -85.8139)
  spline S159 degree 2 poles (-51.2571, -85.8139) (-51.4872, -85.8139) (-51.8535, -85.8949) (-51.9799, -86.0213) knots 0 0 0 1 2 2 2
  spline S160 degree 2 poles (-51.9799, -86.0213) (-52.0966, -86.1315) (-52.2068, -86.4427) (-52.2068, -86.6502) knots 0 0 0 1 2 2 2
  line L246 (-53.672, -83.7782) -> (-53.672, -87.7782)
  line L247 (-53.672, -87.7782) -> (-56.1744, -87.7782)
  line L248 (-56.1744, -87.7782) -> (-56.1744, -87.305)
  line L249 (-56.1744, -87.305) -> (-54.2036, -87.305)
  line L250 (-54.2036, -87.305) -> (-54.2036, -86.2093)
  line L251 (-54.2036, -86.2093) -> (-56.0415, -86.2093)
  line L252 (-56.0415, -86.2093) -> (-56.0415, -85.7361)
  line L253 (-56.0415, -85.7361) -> (-54.2036, -85.7361)
  line L254 (-54.2036, -85.7361) -> (-54.2036, -84.2515)
  line L255 (-54.2036, -84.2515) -> (-56.1744, -84.2515)
  line L256 (-56.1744, -84.2515) -> (-56.1744, -83.7782)
  line L257 (-56.1744, -83.7782) -> (-53.672, -83.7782)
  line L258 (-60.1874, -83.7782) -> (-59.6558, -83.7782)
  line L259 (-59.6558, -83.7782) -> (-59.6558, -87.2239)
  line L260 (-59.6558, -87.2239) -> (-58.612, -84.8803)
  line L261 (-58.612, -84.8803) -> (-58.2879, -84.8803)
  line L262 (-58.2879, -84.8803) -> (-57.2538, -87.2239)
  line L263 (-57.2538, -87.2239) -> (-57.2538, -83.7782)
  line L264 (-57.2538, -83.7782) -> (-56.7579, -83.7782)
  line L265 (-56.7579, -83.7782) -> (-56.7579, -87.7782)
  line L266 (-56.7579, -87.7782) -> (-57.484, -87.7782)
  line L267 (-57.484, -87.7782) -> (-58.4823, -85.5513)
  line L268 (-58.4823, -85.5513) -> (-59.4483, -87.7782)
  line L269 (-59.4483, -87.7782) -> (-60.1874, -87.7782)
  line L270 (-60.1874, -87.7782) -> (-60.1874, -83.7782)
  line L271 (-60.9977, -83.7782) -> (-60.9977, -87.7782)
  line L272 (-60.9977, -87.7782) -> (-63.5002, -87.7782)
  line L273 (-63.5002, -87.7782) -> (-63.5002, -87.305)
  line L274 (-63.5002, -87.305) -> (-61.5293, -87.305)
  line L275 (-61.5293, -87.305) -> (-61.5293, -86.2093)
  line L276 (-61.5293, -86.2093) -> (-63.3673, -86.2093)
  line L277 (-63.3673, -86.2093) -> (-63.3673, -85.7361)
  line L278 (-63.3673, -85.7361) -> (-61.5293, -85.7361)
  line L279 (-61.5293, -85.7361) -> (-61.5293, -84.2515)
  line L280 (-61.5293, -84.2515) -> (-63.5002, -84.2515)
  line L281 (-63.5002, -84.2515) -> (-63.5002, -83.7782)
  line L282 (-63.5002, -83.7782) -> (-60.9977, -83.7782)
  line L283 (-66.9459, -83.7782) -> (-66.3494, -83.7782)
  line L284 (-66.3494, -83.7782) -> (-64.5796, -87.2272)
  line L285 (-64.5796, -87.2272) -> (-64.5796, -83.7782)
  line L286 (-64.5796, -83.7782) -> (-64.0836, -83.7782)
  line L287 (-64.0836, -83.7782) -> (-64.0836, -87.7782)
  line L288 (-64.0836, -87.7782) -> (-64.8389, -87.7782)
  line L289 (-64.8389, -87.7782) -> (-66.4499, -84.6113)
  line L290 (-66.4499, -84.6113) -> (-66.4499, -87.7782)
  line L291 (-66.4499, -87.7782) -> (-66.9459, -87.7782)
  line L292 (-66.9459, -87.7782) -> (-66.9459, -83.7782)
  line L293 (-68.6898, -83.7782) -> (-68.6898, -87.305)
  line L294 (-68.6898, -87.305) -> (-67.3478, -87.305)
  line L295 (-67.3478, -87.305) -> (-67.3478, -87.7782)
  line L296 (-67.3478, -87.7782) -> (-70.5634, -87.7782)
  line L297 (-70.5634, -87.7782) -> (-70.5634, -87.305)
  line L298 (-70.5634, -87.305) -> (-69.2214, -87.305)
  line L299 (-69.2214, -87.305) -> (-69.2214, -83.7782)
  line L300 (-69.2214, -83.7782) -> (-68.6898, -83.7782)
  line L301 (-74.0383, -85.2855) -> (-72.5245, -85.2855)
  line L302 (-72.5245, -85.2855) -> (-72.5245, -85.7717)
  line L303 (-72.5245, -85.7717) -> (-74.0383, -85.7717)
  line L304 (-74.0383, -85.7717) -> (-74.0383, -85.2855)
  line L305 (-77.74, -85.3665) -> (-74.8551, -83.9889)
  line L306 (-74.8551, -83.9889) -> (-74.8551, -84.4654)
  line L307 (-74.8551, -84.4654) -> (-77.0917, -85.5286)
  line L308 (-77.0917, -85.5286) -> (-74.8551, -86.5886)
  line L309 (-74.8551, -86.5886) -> (-74.8551, -87.0651)
  line L310 (-74.8551, -87.0651) -> (-77.74, -85.6874)
  line L311 (-77.74, -85.6874) -> (-77.74, -85.3665)
  point P0 (0, 0)
  constraints: 10 other
extrude "Extrusion3" cut sketch "Sketch3" against normal blind 0.5 contours S0 S1 S2 S3 S4 S5 S6 S7 | L16 L17 S14 S15 S16 S17 S18 S19 L18 L19 S20 S21 S22 S23 S24 L20 L21 | S25 S26 S27 S28 S29 S30 S31 S32 | S39 S40 L22 L23 L24 L25 L26 S41 S42 | S47 S48 S49 S50 L28 L29 S51 S52 S53 L30 L31 S54 S55 | L33 L34 S60 S61 S62 L35 L36 L37 L38 L39 S63 S64 L40 | S65 S66 S67 S68 S69 S70 S71 S72 | L41 L42 L43 L44 L45 L46 L47 L48 L49 L50 L51 L52 | L53 L54 L55 L56 L57 L58 L59 L60 | L61 L62 L63 L64 L65 L66 L67 | L68 L69 L70 L71 | S79 S80 S81 S82 S83 S84 L72 L73 S85 S86 S87 S88 S89 S90 S91 S92 L74 L75 S93 S94 | L76 L77 L78 L79 L80 L81 L82 L83 | L87 L88 L89 L90 L91 L92 | L93 L94 L95 L96 L97 L98 L99 L100 L101 L102 L103 L104 | S95 S96 L105 L106 L107 S97 S98 S99 L108 S100 | L115 L126 L122 | L122 L126 L127 L128 L129 L130 L131 L132 L133 | L115 L116 L117 L118 L119 L120 L121 S109 S110 S111 L122 L126 | L137 L138 L139 L140 L141 L142 L143 L144 | L145 L146 L147 L148 L149 L150 L151 L152 L153 L154 L155 L156 | S116 S117 S118 S119 S120 S121 S122 S123 | L157 L158 L159 L160 L161 L162 L163 L164 L165 L166 | L167 L168 L169 L170 L171 L172 L173 | L174 L175 L176 L177 | L178 L179 L180 L181 | L182 L183 L184 L185 L186 L187 L188 | L189 L190 L191 L192 L193 L194 L195 L196 L197 L198 L199 L200 L201 | L202 L203 L204 L205 L206 L207 L208 L209 L210 L211 L212 L213 | L214 L215 L216 L217 L218 L219 L220 L221 | S130 L225 L226 S131 S132 S133 S134 S135 S136 S137 S138 L227 L228 S139 S140 S141 S142 S143 S144 S145 | S146 S147 L229 L230 L231 S148 S149 S150 S151 L232 L233 L234 S152 S153 | L235 L236 L237 L238 L239 L240 L241 S154 S155 S156 L242 | L246 L247 L248 L249 L250 L251 L252 L253 L254 L255 L256 L257 | L258 L259 L260 L261 L262 L263 L264 L265 L266 L267 L268 L269 L270 | L271 L272 L273 L274 L275 L276 L277 L278 L279 L280 L281 L282 | L283 L284 L285 L286 L287 L288 L289 L290 L291 L292 | L293 L294 L295 L296 L297 L298 L299 L300 | L301 L302 L303 L304 | L305 L306 L307 L308 L309 L310 L311
body "Solid1"
